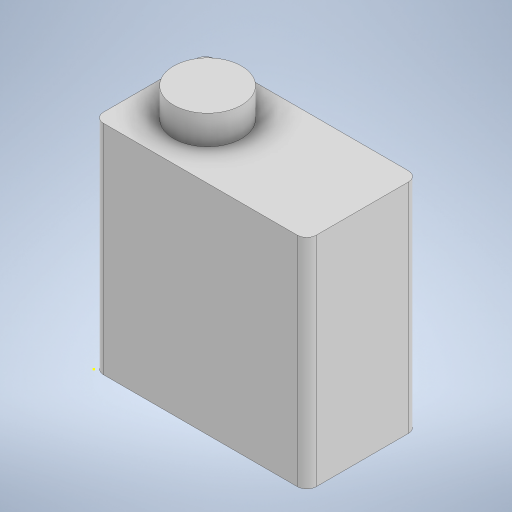
# Autodesk Inventor part: SG-90-servo-motor
Saved by Autodesk Inventor 2023 (Build 270158000, 158)
## iProperties
Created: 2023-01-30
Part Number: SG-90-servo-motor
Material: Generic
Document SubType Name: Modeling
Designer: ringl
Density: 1 g/cm^3
Appearance: Default
Author: ringl
Autodesk Inventor part; units mm, degrees
ref_plane "YZ Plane" through (0, 0, 0) normal (1, 0, 0) x (0, 1, 0)
ref_plane "XZ Plane" through (0, 0, 0) normal (0, 1, 0) x (-1, 0, 0)
ref_plane "XY Plane" through (0, 0, 0) normal (0, 0, 1) x (1, 0, 0)
sketch "Sketch1" plane through (0, 0, 0) normal (0, 1, 0) x (-1, 0, 0)
  line L0 (0, 0) -> (22, 0)
  line L1 (22, 0) -> (22, -11.5)
  line L2 (22, -11.5) -> (0, -11.5)
  line L3 (0, -11.5) -> (0, 0)
  dimension "d0" = 22
  dimension "d1" = 11.5
  constraints: 8 end point, 2 parallel, 1 horizontal, 1 perpendicular
  measures "d0" distance of L1.end L2.end
  measures "d1" distance of L0.end L1.end
extrude "Extrusion1" add sketch "Sketch1" along normal blind 22.5
fillet "Fillet1" radius 1 4 edges at (-22, 11.25, -11.5) (-22, 11.25, 0) (0, 11.25, 0) (0, 11.25, -11.5)
sketch "Sketch2" plane through (-22, 0, -10.5) normal (-1, 0, 0) x (0, 0, 1)
  point P0 (10.5, 0)
sketch "Sketch3" plane through (0, 22.5, 0) normal (0, 1, 0) x (1, 0, 0)
  circle A0 centre (-16, 5.75) radius 3.5
  line L0 (0, 1) -> (0, 10.5) projected
  line L1 (-21, 0) -> (-1, 0) projected
  point P0 (0, 0)
  dimension "d5" = 7
  dimension "d6" = 16
  dimension "d7" = 5.75
  constraints: 1 centre point
  measures "d5" diameter of A0
  measures "d6" distance from line of L0 A0.centre
  measures "d7" distance from line of A0.centre L1
extrude "Extrusion2" add sketch "Sketch3" along normal blind 3
body "Solid1"
